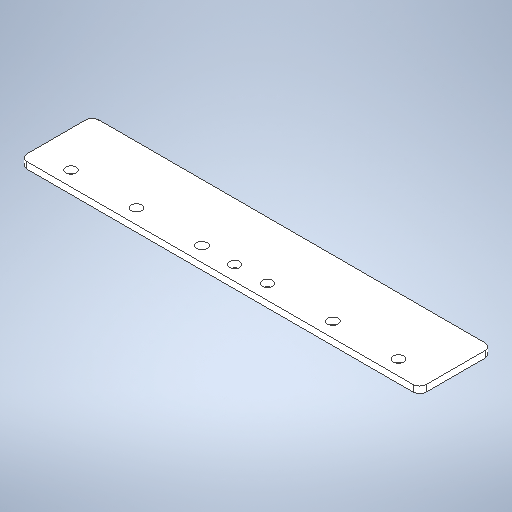
# Autodesk Inventor part: ラインセンサ
Saved by Autodesk Inventor 2026.2 (Build 302298010, 298A)
## iProperties
Created: 2026-05-06
Part Number: ラインセンサ
Material: 一般
Document SubType Name: Modeling
Designer: Yagis
Density: 1 g/cm^3
Appearance: 既定
Author: Yagis
Autodesk Inventor part; units mm, degrees
ref_plane "YZ Plane" through (0, 0, 0) normal (1, 0, 0) x (0, 1, 0)
ref_plane "XZ Plane" through (0, 0, 0) normal (0, 1, 0) x (-1, 0, 0)
ref_plane "XY Plane" through (0, 0, 0) normal (0, 0, 1) x (1, 0, 0)
sketch "スケッチ1" plane through (0, 0, 0) normal (0, 1, 0) x (-1, 0, 0)
  line L0 (0, 0) -> (-122, 0)
  line L1 (-122, 0) -> (-122, -22)
  line L2 (-122, -22) -> (0, -22)
  line L3 (0, -22) -> (0, 0)
  dimension "d0" = 122
  dimension "d1" = 22
  constraints: 8 end point, 2 parallel, 1 horizontal, 1 perpendicular
  measures "d0" distance of L0.start L0.end
  measures "d1" distance of L0.end L1.end
extrude "押し出し1" add sketch "スケッチ1" along normal blind 2
fillet "面フィレット1" radius 2 1 edges at (0, 1, 0)
fillet "面フィレット2" radius 2 1 edges at (0, 1, -22)
fillet "面フィレット3" radius 2 1 edges at (122, 1, -22)
fillet "面フィレット4" radius 2 1 edges at (122, 1, 0)
sketch "スケッチ2" plane through (0, 2, 0) normal (0, 1, 0) x (1, 0, 0)
  line L0 (2, 0) -> (120, 0) projected
  line L1 (0, 20) -> (0, 2) projected
  point P0 (0, 0)
  point P1 (11, 4.5)
  point P2 (31, 4.5)
  point P3 (51, 4.5)
  point P4 (61, 4.5)
  point P5 (71, 4.5)
  point P6 (91, 4.5)
  point P7 (111, 4.5)
  dimension "d8" = 4.5
  dimension "d9" = 11
  dimension "d10" = 20
  dimension "d11" = 20
  dimension "d12" = 10
  dimension "d13" = 10
  dimension "d14" = 20
  dimension "d15" = 20
  constraints: 10 horizontal alignment
  measures "d8" distance from line of L0 point (11, 4.5)
  measures "d9" distance from line of point (11, 4.5) L1
  measures "d10" distance of point (31, 4.5) point (11, 4.5)
  measures "d11" distance of point (51, 4.5) point (31, 4.5)
  measures "d12" distance of point (61, 4.5) point (51, 4.5)
  measures "d13" distance of point (61, 4.5) point (71, 4.5)
  measures "d14" distance of point (91, 4.5) point (71, 4.5)
  measures "d15" distance of point (111, 4.5) point (91, 4.5)
hole "穴1" at (11, 2, -4.5) at (31, 2, -4.5) at (51, 2, -4.5) at (61, 2, -4.5) at (71, 2, -4.5) at (91, 2, -4.5) at (111, 2, -4.5) direction (0, -1, 0) diameter 3.2 depth 8.8 tip angle 118
